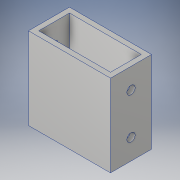
# Autodesk Inventor part: 1x2x2
Saved by Autodesk Inventor 2018 (Build 220112000, 112)
## iProperties
Created: 2018-01-17
Part Number: 1x2x2
Material: Aluminum 6061
Document SubType Name: Modeling
Designer: S-2512711
Density: 2.7 g/cm^3
Appearance: Aluminum - Flat
Mass: 60.837 g
Surface Area: 150.806 cm^2
Volume: 22.5322 cm^3
Author: S-2512711
Autodesk Inventor part; units mm, degrees
ref_plane "YZ Plane" through (0, 0, 0) normal (1, 0, 0) x (0, 1, 0)
ref_plane "XZ Plane" through (0, 0, 0) normal (0, 1, 0) x (-1, 0, 0)
ref_plane "XY Plane" through (0, 0, 0) normal (0, 0, 1) x (1, 0, 0)
sketch "Sketch1" plane through (0, 0, 0) normal (0, 1, 0) x (-1, 0, 0)
  line L0 (0, 0) -> (-50.8, 0)
  line L1 (-50.8, 0) -> (-50.8, -25.4)
  line L2 (-50.8, -25.4) -> (0, -25.4)
  line L3 (0, -25.4) -> (0, 0)
  line L4 (-3.175, -22.225) -> (-47.625, -22.225)
  line L5 (-47.625, -22.225) -> (-47.625, -3.175)
  line L6 (-47.625, -3.175) -> (-3.175, -3.175)
  line L7 (-3.175, -3.175) -> (-3.175, -22.225)
  dimension "d0" = 50.8
  dimension "d1" = 25.4
  dimension "d2" = 3.175
  dimension "d3" = 3.175
  dimension "d4" = 3.175
  dimension "d5" = 3.175
  constraints: 16 end point, 4 parallel, 2 horizontal, 2 perpendicular
  measures "d0" distance of L2.end L1.end
  measures "d1" distance of L0.end L1.end
  measures "d2" distance between parallel lines of L2 L4
  measures "d3" distance between parallel lines of L0 L6
  measures "d4" distance between parallel lines of L1 L5
  measures "d5" distance between parallel lines of L3 L7
extrude "Extrusion1" add sketch "Sketch1" along normal blind 50.8
sketch "Sketch2" plane through (50.8, 0, 0) normal (1, 0, 0) x (0, 0, -1)
  line L0 (0, 0) -> (0, 50.8) projected
  line L1 (0, 0) -> (12.7, 0)
  line L2 (22.225, 0) -> (3.175, 0) projected
  line L3 (12.7, 0) -> (12.7, 12.7)
  line L4 (12.7, 12.7) -> (12.7, 38.1)
  circle A0 centre (12.7, 38.1) radius 2.54
  circle A1 centre (12.7, 12.7) radius 2.54
  dimension "d8" = 12.7
  dimension "d9" = 25.4
  dimension "d10" = 5.08
  constraints: 6 end point, 2 centre point, 2 coincident, 1 midpoint, 1 perpendicular, 1 point on line
  measures "d8" distance of L1.end L3.end
  measures "d9" distance of L3.end L4.end
  measures "d10" diameter of A0
extrude "Extrusion2" cut sketch "Sketch2" against normal blind 61.9125
body "Solid1"
